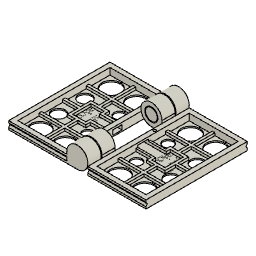
Solar Cell Case Frame v34 (Autodesk Fusion 360 design; units mm, degrees)
Autodesk Fusion 360 part; units mm, degrees
note: some values were not read from the file. Set by a fixed rule: which sketch regions a step uses.
sketch "Sketch1" plane through (0, 0, 0) normal (0, 0, 1) x (1, 0, 0)
  line L0 (0, 0) -> (37.2, 0)
  line L1 (37.2, 0) -> (37.2, 70)
  line L2 (37.2, 70) -> (0, 70)
  line L3 (0, 70) -> (0, 0)
  line L4 (-3.5, -3.5) -> (40.7, -3.5)
  line L5 (40.7, -3.5) -> (40.7, 73.5)
  line L6 (40.7, 73.5) -> (-3.5, 73.5)
  line L7 (-3.5, 73.5) -> (-3.5, -3.5)
  line L8 (60.2, 0) -> (97.4, 0)
  line L9 (97.4, 0) -> (97.4, 70)
  line L10 (97.4, 70) -> (60.2, 70)
  line L11 (60.2, 70) -> (60.2, 0)
  line L12 (56.7, -3.5) -> (100.9, -3.5)
  line L13 (100.9, -3.5) -> (100.9, 73.5)
  line L14 (100.9, 73.5) -> (56.7, 73.5)
  line L15 (56.7, 73.5) -> (56.7, -3.5)
  line L16 (13.6, 42) -> (23.6, 42)
  line L17 (23.6, 42) -> (23.6, 28)
  line L18 (23.6, 28) -> (13.6, 28)
  line L19 (13.6, 28) -> (13.6, 42)
  line L20 (23.6, 38.5) -> (40.7, 38.5)
  line L21 (40.7, 38.5) -> (40.7, 31.5)
  line L22 (40.7, 31.5) -> (23.6, 31.5)
  line L23 (23.6, 31.5) -> (23.6, 38.5)
  line L24 (73.8, 42) -> (83.8, 42)
  line L25 (83.8, 42) -> (83.8, 28)
  line L26 (83.8, 28) -> (73.8, 28)
  line L27 (73.8, 28) -> (73.8, 42)
  line L28 (73.8, 39) -> (56.7, 39)
  line L29 (56.7, 39) -> (56.7, 31)
  line L30 (56.7, 31) -> (73.8, 31)
  line L31 (73.8, 31) -> (73.8, 39)
  line L32 (0, 52) -> (37.2, 52)
  line L33 (0, 18) -> (37.2, 18)
  line L34 (0, 16) -> (37.2, 16)
  line L35 (0, 54) -> (37.2, 54)
  line L36 (17.6, 70) -> (17.6, 42)
  line L37 (19.6, 70) -> (19.6, 42)
  line L38 (17.6, 28) -> (17.6, 0)
  line L39 (19.6, 28) -> (19.6, 0)
  line L40 (0, 36) -> (13.6, 36)
  line L41 (0, 34) -> (13.6, 34)
  line L42 (60.2, 54) -> (97.4, 54)
  line L43 (60.2, 52) -> (97.4, 52)
  line L44 (83.8, 36) -> (97.4, 36)
  line L45 (83.8, 34) -> (97.4, 34)
  line L46 (77.8, 70) -> (77.8, 42)
  line L47 (77.8, 28) -> (77.8, 0)
  line L48 (60.2, 18) -> (97.4, 18)
  line L49 (60.2, 16) -> (97.4, 16)
  line L50 (79.8, 70) -> (79.8, 42)
  line L51 (79.8, 28) -> (79.8, 0)
  line L52 (25.6, 26) -> (11.6, 26)
  line L53 (11.6, 26) -> (11.6, 44)
  line L54 (11.6, 44) -> (25.6, 44)
  line L55 (25.6, 44) -> (25.6, 26)
  line L56 (40.7, 29.5) -> (25.6, 29.5)
  line L57 (25.6, 40.5) -> (40.7, 40.5)
  line L58 (85.8, 26) -> (71.8, 26)
  line L59 (71.8, 26) -> (71.8, 44)
  line L60 (71.8, 44) -> (85.8, 44)
  line L61 (85.8, 44) -> (85.8, 26)
  line L62 (56.7, 40.5) -> (71.8, 40.5)
  line L63 (56.7, 29.5) -> (71.8, 29.5)
  line L64 (-3.5, 73.5) -> (100.9, 73.5)
  line L65 (100.9, 73.5) -> (100.9, -3.5)
  line L66 (100.9, -3.5) -> (-3.5, -3.5)
  line L67 (-3.5, -3.5) -> (-3.5, 73.5)
  dimension "d1" = 37.2
  dimension "d2" = 70
  dimension "d3" = 3.5
  dimension "d18" = 37.2
  dimension "d19" = 70
  dimension "d20" = 3.5
  dimension "d21" = 16
  dimension "d72" = 10
  dimension "d73" = 14
  dimension "d74" = 7
  dimension "d75" = 3.5
  dimension "d76" = 28
  dimension "d77" = 13.6
  dimension "d78" = 10
  dimension "d79" = 14
  dimension "d80" = 8
  dimension "d81" = 28
  dimension "d82" = 13.6
  dimension "d85" = 2
  dimension "d86" = 2
  dimension "d87" = 2
  dimension "d88" = 2
  dimension "d89" = 2
  dimension "d90" = 17.6
  dimension "d91" = 16
  dimension "d92" = 16
  dimension "d93" = 34
  dimension "d94" = 17.6
  dimension "d95" = 2
  dimension "d96" = -2
  dimension "d98" = 2
  dimension "d99" = 2
  dimension "d100" = -2
  constraint horizontal L0
  constraint vertical L1
  constraint horizontal L2
  constraint vertical L3
  constraint coincident L0.start L3.end
  constraint horizontal L8
  constraint vertical L9
  constraint horizontal L10
  constraint vertical L11
  constraint collinear L4 L12
  constraint horizontal L16
  constraint vertical L17
  constraint horizontal L18
  constraint vertical L19
  constraint horizontal L20
  constraint vertical L21
  constraint horizontal L22
  constraint vertical L23
  constraint coincident L17 L20.start
  constraint coincident L5 L20.end
  constraint horizontal L24
  constraint vertical L25
  constraint horizontal L26
  constraint vertical L27
  constraint horizontal L28
  constraint vertical L29
  constraint horizontal L30
  constraint vertical L31
  constraint coincident L15 L29.end
  constraint coincident L27 L28.start
  constraint coincident L3 L32.start
  constraint coincident L1 L32.end
  constraint perpendicular L1 L32
  constraint coincident L3 L33.start
  constraint coincident L1 L33.end
  constraint perpendicular L1 L33
  constraint coincident L3 L34.start
  constraint coincident L1 L34.end
  constraint perpendicular L1 L34
  constraint coincident L1 L35.end
  constraint perpendicular L1 L35
  constraint coincident L2 L36.start
  constraint perpendicular L2 L36
  constraint coincident L2 L37.start
  constraint coincident L16 L37.end
  constraint perpendicular L16 L37
  constraint coincident L18 L38.start
  constraint coincident L0 L38.end
  constraint perpendicular L0 L38
  constraint coincident L18 L39.start
  constraint perpendicular L18 L39
  constraint coincident L3 L40.start
  constraint coincident L19 L40.end
  constraint perpendicular L19 L40
  constraint coincident L3 L41.start
  constraint coincident L19 L41.end
  constraint perpendicular L19 L41
  constraint vertical L36.end L38.start
  constraint coincident L11 L42.start
  constraint coincident L9 L42.end
  constraint perpendicular L9 L42
  constraint coincident L11 L43.start
  constraint coincident L9 L43.end
  constraint perpendicular L9 L43
  constraint coincident L25 L44.start
  constraint coincident L9 L44.end
  constraint perpendicular L9 L44
  constraint coincident L25 L45.start
  constraint coincident L9 L45.end
  constraint perpendicular L9 L45
  constraint coincident L10 L46.start
  constraint coincident L24 L46.end
  constraint perpendicular L24 L46
  constraint coincident L26 L47.start
  constraint coincident L8 L47.end
  constraint perpendicular L8 L47
  constraint coincident L11 L48.start
  constraint coincident L9 L48.end
  constraint perpendicular L9 L48
  constraint coincident L11 L49.start
  constraint coincident L9 L49.end
  constraint perpendicular L9 L49
  constraint horizontal L40.end L44.start
  constraint horizontal L41.end L45.start
  constraint horizontal L35.end L42.start
  constraint horizontal L32.end L43.start
  constraint horizontal L33.end L48.start
  constraint horizontal L34.end L49.start
  constraint vertical L46.end L47.start
  constraint coincident L10 L50.start
  constraint coincident L24 L50.end
  constraint perpendicular L24 L50
  constraint coincident L26 L51.start
  constraint coincident L8 L51.end
  constraint perpendicular L8 L51
  constraint vertical L50.end L51.start
  constraint coincident L5 L56.start
  constraint coincident L55 L56.end
  constraint perpendicular L55 L56
  constraint coincident L55 L57.start
  constraint coincident L5 L57.end
  constraint perpendicular L5 L57
  constraint coincident L15 L62.start
  constraint coincident L59 L62.end
  constraint perpendicular L59 L62
  constraint horizontal L57.end L62.start
  constraint coincident L15 L63.start
  constraint coincident L59 L63.end
  constraint perpendicular L59 L63
  constraint horizontal L56.start L63.start
  constraint horizontal L64
  constraint vertical L65
  constraint horizontal L66
  constraint vertical L67
  measures "d1" distance of L0.start L0.end
  measures "d2" distance of L0.start L2.end
  measures "d18" distance of L8.start L8.end
  measures "d19" distance of L8.start L10.end
  measures "d21" distance of L5 L15
  measures "d72" distance of L16.start L16.end
  measures "d73" distance of L16.start L18.end
  measures "d74" distance of L20.start L22.end
  measures "d75" distance of L16 L20
  measures "d76" distance of L2 L16
  measures "d77" distance of L3 L19
  measures "d78" distance of L24.start L24.end
  measures "d79" distance of L24.start L26.end
  measures "d80" distance of L28.start L30.end
  measures "d81" distance of L10 L24
  measures "d82" distance of L9 L25
  measures "d85" distance of L32 L35
  measures "d86" distance of L40 L41
  measures "d87" distance of L33 L34
  measures "d88" distance of L38 L39
  measures "d89" distance of L36 L37
  measures "d90" distance of L3 L36
  measures "d91" distance of L2 L35
  measures "d92" distance of L0 L34
  measures "d93" distance of L2 L40
  measures "d94" distance of L9 L50
  measures "d95" distance of L46 L50
  measures "d98" distance of L22 L56
  measures "d99" distance of L20 L57
extrude "Extrude13" add sketch "Sketch1" along normal blind 1 contours L0 L3 L34 L38 | L0 L1 L34 L39 | L3 L33 L38 L41 L52 L53 | L1 L33 L39 L52 L55 L56 | L3 L32 L36 L40 L53 L54 | L16 L17 L18 L19 L23 | L2 L3 L35 L36 | L1 L20 L22 L55 | L1 L5 L20 L21 L22 | L1 L32 L37 L54 L55 L57 | L17 L20 L22 L23 L55 | L1 L2 L35 L37 | L11 L15 L28 L29 L30 | L11 L47 L48 L58 L59 L63 | L11 L28 L30 L59 | L27 L28 L30 L31 L59 | L8 L11 L47 L49 | L11 L43 L46 L59 L60 L62 | L24 L25 L26 L27 L31 | L9 L45 L48 L51 L58 L61 | L8 L9 L49 L51 | L10 L11 L42 L46 | L9 L43 L44 L50 L60 L61 | L9 L10 L42 L50 makes body 1 at (16.9333, 36.1667, 0) makes body 2 at (33.3333, 24.5, 0) makes body 3 at (31.3333, 59.3333, 0) makes body 4 at (11.7333, 59.3333, 0) makes body 5 at (3.8667, 26, 0) makes body 6 at (25.4667, 5.3333, 0) makes body 7 at (33.3333, 45.5, 0) makes body 8 at (3.8667, 44, 0) makes body 9 at (5.8667, 5.3333, 0) makes body 10 at (64.0667, 45.5, 0) makes body 11 at (93.5333, 26, 0) makes body 12 at (64.0667, 24.5, 0) makes body 13 at (66.0667, 64.6667, 0) makes body 14 at (93.5333, 44, 0) makes body 15 at (85.6667, 10.6667, 0) makes body 16 at (66.0667, 10.6667, 0) makes body 17 at (80.4667, 33.6667, 0) makes body 18 at (85.6667, 64.6667, 0)
extrude "Extrude5" add sketch "Sketch1" along normal blind 6 contours L0 L1 L2 L3 L4 L5 L6 L7 L56 L57 L64 L66 L67 | L1 L5 L22 L56 | L1 L5 L20 L57 | L8 L9 L10 L11 L12 L13 L14 L15 L62 L63 L64 L65 L66 | L11 L15 L30 L63 | L11 L15 L28 L62 bodies 10 1 17 2 11 12 13 14 15 16 18 3 4 5 6 7 8 9
extrude "Extrude1" add sketch "Sketch1" along normal blind 3 contours L0 L34 L38 L39 | L3 L33 L34 L38 | L33 L34 L38 L39 | L1 L33 L34 L39 | L33 L38 L39 L52 | L3 L40 L41 L53 | L18 L19 L38 L41 L52 L53 | L18 L38 L39 L52 | L19 L40 L41 L53 | L17 L18 L22 L39 L52 L55 | L3 L32 L35 L36 | L16 L19 L36 L40 L53 L54 | L1 L22 L55 L56 | L32 L35 L36 L37 | L32 L36 L37 L54 | L2 L35 L36 L37 | L1 L32 L35 L37 | L16 L36 L37 L54 | L1 L20 L55 L57 | L16 L17 L20 L37 L54 L55 | L11 L30 L59 L63 | L11 L47 L48 L49 | L26 L27 L30 L47 L58 L59 | L11 L28 L59 L62 | L47 L48 L49 L51 | L47 L48 L51 L58 | L24 L27 L28 L46 L59 L60 | L8 L47 L49 L51 | L26 L47 L51 L58 | L9 L48 L49 L51 | L11 L42 L43 L46 | L25 L26 L45 L51 L58 L61 | L42 L43 L46 L50 | L43 L46 L50 L60 | L9 L44 L45 L61 | L10 L42 L46 L50 | L9 L42 L43 L50 | L24 L46 L50 L60 | L25 L44 L45 L61 | L24 L25 L44 L50 L60 L61 bodies 10 1
sketch "Sketch2" plane through (0, -3.5, 0) normal (0, -1, 0) x (1, 0, 0)
  line L0 (-3.5, 0) -> (40.7, 0)
  line L1 (40.7, 0) -> (40.7, 6)
  line L2 (40.7, 6) -> (-3.5, 6)
  line L3 (-3.5, 6) -> (-3.5, 0)
  line L4 (40.7, 0) -> (40.7, 8)
  line L5 (40.7, 0) -> (48.7, 0)
  arc A0 (48.7, 0) -> (40.7, 8) centre (48.7, 8) ccw
  line L6 (-3.5, 0) -> (40.7, 0)
  line L7 (40.7, 0) -> (40.7, 6)
  line L8 (40.7, 6) -> (-3.5, 6)
  line L9 (-3.5, 6) -> (-3.5, 0)
  dimension "d8" = 8
  dimension "d9" = 8
  constraint coincident L0.end L1.start
  constraint perpendicular L2 L4
  constraint perpendicular L4 L5
  constraint tangent L5 A0
  measures "d8" distance of L0.end L4.end
  measures "d9" distance of L0.end L5.end
extrude "Extrude3" add sketch "Sketch2" against normal blind 10 contours L1 L4 L5 A0 L7 bodies 1
sketch "Sketch3" plane through (0, 73.5, 0) normal (0, 1, 0) x (-1, 0, 0)
  line L0 (-40.7, 0) -> (3.5, 0)
  line L1 (3.5, 0) -> (3.5, 6)
  line L2 (3.5, 6) -> (-40.7, 6)
  line L3 (-40.7, 6) -> (-40.7, 0)
  line L4 (-40.7, 0) -> (-48.7, 0)
  line L5 (-40.7, 0) -> (-40.7, 8)
  arc A0 (-40.7, 8) -> (-48.7, 0) centre (-48.7, 8) ccw
  line L6 (-40.7, 0) -> (3.5, 0)
  line L7 (3.5, 0) -> (3.5, 6)
  line L8 (3.5, 6) -> (-40.7, 6)
  line L9 (-40.7, 6) -> (-40.7, 0)
  dimension "d13" = 8
  dimension "d14" = 8
  constraint coincident L0.start L3.end
  constraint perpendicular L3 L4
  constraint perpendicular L2 L5
  constraint tangent L4 A0
  measures "d13" distance of L0.start L4.end
  measures "d14" distance of L0.start L5.end
extrude "Extrude4" add sketch "Sketch3" against normal blind 10 contours L3 L4 L5 A0 L9 bodies 1
sketch "Sketch13" plane through (0, 6.5, 0) normal (0, 1, 0) x (1, 0, 0)
  line L0 (-3.5, 0) -> (48.7, 0)
  circle A0 centre (48.7, -8) radius 4.5
  arc A1 (40.7, -8) -> (48.7, 0) centre (48.7, -8) ccw
  line L1 (48.7, 0) -> (40.7, 0)
  line L2 (40.7, 0) -> (40.7, -6)
  line L3 (40.7, -6) -> (40.7, -8)
  arc A2 (40.7, -8) -> (48.7, 0) centre (48.7, -8) ccw
  line L4 (48.7, 0) -> (40.7, 0)
  line L5 (40.7, 0) -> (40.7, -6)
  line L6 (40.7, -6) -> (40.7, -8)
  dimension "d137" = 9
  constraint coincident A0.centre A1.centre
  measures "d137" diameter of A0
extrude "Extrude17" add sketch "Sketch13" along normal blind 10.7 contours A0 bodies 1
sketch "Sketch14" plane through (0, 63.5, 0) normal (0, -1, 0) x (1, 0, 0)
  arc A0 (48.7, 0) -> (40.7, 8) centre (48.7, 8) ccw
  line L0 (40.7, 8) -> (40.7, 6)
  line L1 (40.7, 6) -> (40.7, 0)
  line L2 (40.7, 0) -> (48.7, 0)
  circle A1 centre (48.7, 8) radius 4.5
  dimension "d141" = 9
  constraint concentric A0 A1
  measures "d141" diameter of A1
extrude "Extrude18" add sketch "Sketch14" along normal blind 10.7 contours A1 bodies 1
ref_plane "WorkPlane1" through (48.7, 17.2, 8) normal (0, 1, 0) x (1, 0, 0)
sketch "Sketch16" plane through (48.7, 17.2, 8) normal (0, 1, 0) x (1, 0, 0)
  line L0 (8, 8) -> (8, 0)
  line L1 (8, 8) -> (0, 8)
  arc A0 (0, 8) -> (8, 0) centre (0, 0) ccw
  circle A1 centre (0, 0) radius 5
  dimension "d148" = 8
  dimension "d149" = 8
  dimension "d150" = 10
  constraint vertical L0
  constraint perpendicular L0 L1
  constraint tangent L0 A0
  constraint concentric A0 A1
  measures "d148" distance of L0.start L0.end
  measures "d149" distance of L0.start L1.end
  measures "d150" diameter of A1
extrude "Extrude19" add sketch "Sketch16" against normal blind 10 bodies 10
ref_plane "WorkPlane2" through (48.7, 52.8, 8) normal (0, -1, 0) x (1, 0, 0)
sketch "Sketch18" plane through (48.7, 52.8, 8) normal (0, -1, 0) x (1, 0, 0)
  circle A0 centre (0, 0) radius 5
  line L0 (8, -8) -> (0, -8)
  line L1 (8, -8) -> (8, 0)
  arc A1 (8, 0) -> (0, -8) centre (0, 0) ccw
  dimension "d159" = 10
  dimension "d160" = 8
  dimension "d161" = 8
  constraint coincident A0.centre A1.centre
  constraint horizontal L0
  constraint perpendicular L0 L1
  constraint tangent L1 A1
  measures "d159" diameter of A0
  measures "d160" distance of L0.start L0.end
  measures "d161" distance of L0.start L1.end
extrude "Extrude20" add sketch "Sketch18" against normal blind 10 bodies 10
sketch "Sketch9" plane through (-3.5, 0, 0) normal (-1, 0, 0) x (0, -1, 0)
  line L0 (-73.5, 0) -> (3.5, 0)
  line L1 (3.5, 0) -> (3.5, 6)
  line L2 (3.5, 6) -> (-73.5, 6)
  line L3 (-73.5, 6) -> (-73.5, 0)
  line L4 (-73.5, 4.5) -> (-72.5, 3)
  line L5 (-72.5, 3) -> (-73.5, 1.5)
  line L6 (3.5, 4.5) -> (2.5, 3)
  line L7 (2.5, 3) -> (3.5, 1.5)
  line L8 (-73.5, 0) -> (3.5, 0)
  line L9 (3.5, 0) -> (3.5, 6)
  line L10 (3.5, 6) -> (-73.5, 6)
  line L11 (-73.5, 6) -> (-73.5, 0)
  dimension "d45" = 1
  dimension "d46" = 1
  dimension "d47" = 3
  dimension "d49" = 1.5
  dimension "d127" = 1.5
  constraint coincident L3 L4.start
  constraint coincident L3 L5.end
  constraint coincident L1 L6.start
  constraint coincident L1 L7.end
  constraint horizontal L5.end L7.end
  constraint horizontal L4.start L6.start
  constraint horizontal L4.end L6.end
  measures "d45" distance of L3 L4.end
  measures "d46" distance of L1 L6.end
  measures "d47" distance of L4.start L5.end
  measures "d49" vertical distance of L4.start L4.end
  measures "d127" distance of L4.start L2.end
extrude "Extrude11" cut sketch "Sketch9" against normal blind 44.2 contours L3 L4 L5 L11 | L1 L6 L7 L9 bodies 1
sketch "Sketch10" plane through (100.9, 0, 0) normal (1, 0, 0) x (0, 1, 0)
  line L0 (-3.5, 0) -> (73.5, 0)
  line L1 (73.5, 0) -> (73.5, 6)
  line L2 (73.5, 6) -> (-3.5, 6)
  line L3 (-3.5, 6) -> (-3.5, 0)
  line L4 (-3.5, 4.5) -> (-2.5, 3)
  line L5 (-2.5, 3) -> (-3.5, 1.5)
  line L6 (73.5, 4.5) -> (72.5, 3)
  line L7 (72.5, 3) -> (73.5, 1.5)
  line L8 (-3.5, 4.5) -> (-3.5, 1.5)
  dimension "d54" = 1
  dimension "d55" = 1
  dimension "d56" = 3
  dimension "d57" = 5
  dimension "d58" = 1.5
  dimension "d59" = 1.5
  constraint coincident L3 L4.start
  constraint coincident L3 L5.end
  constraint coincident L1 L6.start
  constraint coincident L1 L7.end
  constraint horizontal L5.end L7.end
  constraint horizontal L4.start L6.start
  constraint horizontal L4.end L6.end
  measures "d54" horizontal distance of L4.end L5.end
  measures "d55" distance of L1 L6.end
  measures "d56" distance of L4.start L5.end
  measures "d58" distance of L2.end L4.start
  measures "d59" vertical distance of L4.start L4.end
extrude "Extrude12" cut sketch "Sketch10" against normal blind 44.2 contours L3 L4 L5 L8 | L1 L6 L7 bodies 10
hole "Hole1" at (58.45, 45.5, 6) direction (0, 0, -1) diameter 2 depth 4 tip angle 118 bodies 10
hole "Hole2" at (38.95, 24.5, 6) direction (0, 0, -1) diameter 2 depth 4 tip angle 118 bodies 1
sketch "Sketch11" plane through (0, 0, 0) normal (0, 0, 1) x (1, 0, 0)
  circle A0 centre (88.4, 8) radius 7
  circle A1 centre (69.2, 8) radius 7
  circle A2 centre (88.4, 62) radius 7
  circle A3 centre (69.2, 62) radius 7
  circle A4 centre (9, 62) radius 7
  circle A5 centre (28.2, 62) radius 7
  circle A6 centre (9, 8) radius 7
  circle A7 centre (28.2, 8) radius 7
  circle A8 centre (6, 45) radius 5
  circle A9 centre (30.2, 47) radius 4
  circle A10 centre (6, 25) radius 5
  circle A11 centre (30.2, 23) radius 4
  circle A12 centre (67.2, 47) radius 4
  circle A13 centre (91.4, 45) radius 5
  circle A14 centre (67.2, 23) radius 4
  circle A15 centre (91.4, 25) radius 5
  line L0 (0, 70) -> (0, 0)
  line L1 (37.2, 0) -> (37.2, 70)
  line L2 (60.2, 70) -> (60.2, 0)
  line L3 (97.4, 0) -> (97.4, 70)
  dimension "d101" = 14
  dimension "d102" = 14
  dimension "d103" = 14
  dimension "d104" = 14
  dimension "d105" = 14
  dimension "d106" = 14
  dimension "d107" = 14
  dimension "d108" = 14
  dimension "d109" = 10
  dimension "d110" = 8
  dimension "d111" = 10
  dimension "d112" = 8
  dimension "d113" = 8
  dimension "d114" = 10
  dimension "d115" = 8
  dimension "d116" = 10
  dimension "d117" = 9
  dimension "d118" = 9
  dimension "d119" = 9
  dimension "d120" = 9
  dimension "d121" = 6
  dimension "d122" = 6
  dimension "d123" = 7
  dimension "d124" = 7
  constraint horizontal A4.centre A5.centre
  constraint horizontal A3.centre A5.centre
  constraint horizontal A2.centre A3.centre
  constraint vertical A8.centre A10.centre
  constraint horizontal A6.centre A7.centre
  constraint horizontal A0.centre A1.centre
  constraint vertical A13.centre A15.centre
  constraint vertical A12.centre A14.centre
  constraint vertical A9.centre A11.centre
  constraint horizontal A11.centre A14.centre
  constraint horizontal A9.centre A12.centre
  constraint horizontal A8.centre A13.centre
  constraint horizontal A10.centre A15.centre
  constraint vertical A4.centre A6.centre
  constraint vertical A5.centre A7.centre
  constraint vertical A1.centre A3.centre
  constraint vertical A0.centre A2.centre
  measures "d101" diameter of A0
  measures "d102" diameter of A1
  measures "d103" diameter of A2
  measures "d104" diameter of A3
  measures "d105" diameter of A4
  measures "d106" diameter of A5
  measures "d107" diameter of A6
  measures "d108" diameter of A7
  measures "d109" diameter of A8
  measures "d110" diameter of A9
  measures "d111" diameter of A10
  measures "d112" diameter of A11
  measures "d113" diameter of A12
  measures "d114" diameter of A13
  measures "d115" diameter of A14
  measures "d116" diameter of A15
  measures "d117" distance of A4.centre L0
  measures "d118" distance of A5.centre L1
  measures "d119" distance of A3.centre L2
  measures "d120" distance of A2.centre L3
  measures "d121" distance of A13.centre L3
  measures "d122" distance of A8.centre L0
  measures "d123" distance of A9.centre L1
  measures "d124" distance of A12.centre L2
extrude "Extrude14" cut sketch "Sketch11" along normal blind 4 bodies 10 1
sketch "Sketch12" plane through (0, 0, 0) normal (0, 0, -1) x (1, 0, 0)
  circle A0 centre (91.4, -25) radius 5
  circle A1 centre (88.4, -62) radius 7
  circle A2 centre (91.4, -45) radius 5
  circle A3 centre (88.4, -8) radius 7
  circle A4 centre (67.2, -23) radius 4
  circle A5 centre (69.2, -62) radius 7
  circle A6 centre (67.2, -47) radius 4
  circle A7 centre (69.2, -8) radius 7
  line L0 (56.7, -62.8) -> (56.7, -73.5)
  line L1 (56.7, -73.5) -> (100.9, -73.5)
  line L2 (100.9, -73.5) -> (100.9, 3.5)
  line L3 (100.9, 3.5) -> (56.7, 3.5)
  line L4 (12.5158, -27.0304) -> (12.5158, -45.4562) construction
  line L5 (12.5158, -45.4562) -> (20.5158, -45.4562) construction
  line L6 (20.5158, -45.4562) -> (20.5158, -27.0304) construction
  line L7 (20.5158, -27.0304) -> (12.5158, -27.0304) construction
  line L8 (78.8659, -28.3369) -> (78.8659, -43.5947) construction
  line L9 (78.8659, -43.5947) -> (86.8659, -43.5947) construction
  line L10 (86.8659, -43.5947) -> (86.8659, -28.3369) construction
  line L11 (86.8659, -28.3369) -> (78.8659, -28.3369) construction
  line L12 (19.1648, -29.0069) -> (19.1648, -44.2647) construction
  line L13 (19.1648, -44.2647) -> (27.1648, -44.2647) construction
  line L14 (27.1648, -44.2647) -> (27.1648, -29.0069) construction
  line L15 (27.1648, -29.0069) -> (19.1648, -29.0069) construction
  line L16 (72.1499, -26.9634) -> (72.1499, -45.3892) construction
  line L17 (72.1499, -45.3892) -> (80.1499, -45.3892) construction
  line L18 (80.1499, -45.3892) -> (80.1499, -26.9634) construction
  line L19 (80.1499, -26.9634) -> (72.1499, -26.9634) construction
  line L20 (56.7, -17.2) -> (56.7, -52.8)
  line L21 (56.7, -52.8) -> (48.7, -52.8)
  line L22 (48.7, -52.8) -> (48.7, -62.8)
  line L23 (48.7, -62.8) -> (56.7, -62.8)
  line L24 (56.7, 3.5) -> (56.7, -7.2)
  line L25 (56.7, -7.2) -> (48.7, -7.2)
  line L26 (48.7, -7.2) -> (48.7, -17.2)
  line L27 (48.7, -17.2) -> (56.7, -17.2)
  text T0 "Solar" font "Arial" height 8 align ink ink in box 0 x 0 at (12.5358, -27.0404) x (0, -1) y (1, 0) spacing 1 height is em
  text T1 "Ferg" font "Arial" height 8 align ink ink in box 0 x 0 at (78.8859, -28.3469) x (0, -1) y (1, 0) spacing 1 height is em
  text T2 "Ferg" font "Arial" height 8 align ink ink in box 0 x 0 at (19.1848, -29.0169) x (0, -1) y (1, 0) spacing 1 height is em
  text T3 "Solar" font "Arial" height 8 align ink ink in box 0 x 0 at (72.1699, -26.9734) x (0, -1) y (1, 0) spacing 1 height is em
  constraint perpendicular L4 L5
  constraint parallel L4 L6
  constraint parallel L5 L7
  constraint perpendicular L8 L9
  constraint parallel L8 L10
  constraint parallel L9 L11
  constraint perpendicular L12 L13
  constraint parallel L12 L14
  constraint parallel L13 L15
  constraint perpendicular L16 L17
  constraint parallel L16 L18
  constraint parallel L17 L19
extrude "Extrude16" cut sketch "Sketch12" against normal blind 0.5 text T0 T2 T3 T1 bodies 10 1
ref_plane "WorkPlane3" through (18.6, 35, 4.5) normal (0, 0, 1) x (1, 0, 0)
split_face "SplitFace1" 2 faces at (57.8667, 31, 3.3333) (39.5333, 31.5, 3.3333) by plane through (18.6, 35, 4.5) normal (0, 0, 1) on bodies 1 10
move_face "OffsetFaces1" offset 9 2 faces at (57.8667, 31, 5) (39.5333, 31.5, 5) on bodies 1 10
sketch "Sketch8" plane through (0, 0, 0) normal (0, 0, 1) x (1, 0, 0)
  line L0 (63, 78) -> (-6, 78)
  line L1 (-6, -5) -> (63, -5)
  line L2 (63, -5) -> (63, 78)
  line L3 (-6, -5) -> (-6, 6)
  line L4 (-6, 6) -> (34, 7)
  line L5 (34, 7) -> (32.5121, 66.5164)
  line L6 (32.5121, 66.5164) -> (-6, 65.5536)
  line L7 (-6, 65.5536) -> (-6, 78)
  constraint horizontal L0
  constraint horizontal L1
  constraint vertical L2
  constraint perpendicular L1 L3
  constraint perpendicular L4 L5
  constraint perpendicular L5 L6
  constraint perpendicular L0 L7
split "Split1" [suppressed]
combine "Combine1" [suppressed] in component "Component"
hole "Hole3" [suppressed]
hole "Hole2'" [suppressed] in component "Component"
combine "Combine1'" [suppressed] in component "Component'"
component "Component'" placed x (1, 0, 0) y (0, 1, 0) z (0, 0, 1) at (0, 0, 0)
equation "d9 = d8"
equation "d14 = d13"
equation "d18 = d1"
equation "d19 = d2"
equation "d20 = d3"
equation "d46 = d45"
equation "d49 = d47 / 2"
equation "d55 = d54"
equation "d58 = ( 6.00 mm - d56 ) / 2"
equation "d59 = d56 / 2"
equation "d75 = ( d73 - d74 ) / 2"
equation "d76 = ( d2 - d73 ) / 2"
equation "d77 = ( d1 - d72 ) / 2"
equation "d81 = ( d19 - d79 ) / 2"
equation "d82 = ( d18 - d78 ) / 2"
equation "d86 = d85"
equation "d87 = d85"
equation "d88 = d85"
equation "d89 = d85"
equation "d90 = ( d1 - d89 ) / 2"
equation "d91 = ( d2 - 3 * d85 ) / 4"
equation "d92 = d91"
equation "d93 = ( d2 - d85 ) / 2"
equation "d94 = d90"
equation "d95 = d85"
equation "d118 = d117"
equation "d119 = d117"
equation "d120 = d117"
equation "d121 = d122"
equation "d124 = d123"
equation "d127 = ( 6 mm - d47 ) / 2"
